Autodesk Inventor part; units mm, degrees
(part 2 of 2)
extrude "Extrusion65" cut sketch "Sketch70" against normal blind 1.5 contours L6 L7 L8 L0 | L4 L17 L14 L15
sketch "Sketch71" plane through (0, 1.5, 0) normal (0, 1, 0) x (1, 0, 0)
  line L0 (6.4642, -4.9) -> (13.4642, -4.9) projected
  line L1 (-3.6078, -4.9) -> (3.3922, -4.9) projected
  line L2 (-3.6078, -3.9) -> (3.3922, -3.9)
  line L3 (6.4642, -3.9) -> (13.4642, -3.9)
  line L4 (-3.4042, -4.9) -> (3.3922, -4.9)
  line L5 (13.4642, -4.9) -> (6.4642, -4.9)
  line L6 (6.4642, -4.9) -> (6.4642, -3.9)
  line L7 (13.4642, -4.9) -> (13.4642, -3.9)
  line L8 (6.4642, -4.9) -> (6.4642, -3.9)
  line L9 (13.4642, -4.9) -> (6.4642, -4.9)
  line L10 (3.3922, -3.9) -> (3.3922, -4.9)
  line L11 (3.3922, -4.9) -> (-3.6078, -4.9)
  line L12 (-3.6078, -4.9) -> (-3.6078, -3.9)
  point P0 (3.3922, -22.9)
  point P1 (0, 0)
  dimension "d349" = 7
  dimension "d351" = 7
  constraints: 22 end point, 4 collinear, 1 point on line
  measures "d349" distance of L2.start L2.end
  measures "d351" distance of L3.start L3.end
extrude "Extrusion66" cut sketch "Sketch71" against normal blind 1.5
sketch "Sketch75" plane through (0, 1.5, 0) normal (0, 1, 0) x (1, 0, 0)
  line L0 (-14, 20) -> (14, 20) projected
  line L1 (-14, 20) -> (0, 20)
  line L2 (0, 20) -> (0, 11.7)
  line L3 (0, 11.7) -> (-11.6, 11.7)
  line L4 (-11.6, 11.7) -> (12, 11.7)
  line L5 (12, 11.7) -> (12, -0.7)
  line L6 (12, -0.7) -> (-11.6, -0.7)
  line L7 (-11.6, -0.7) -> (-11.6, 11.7)
  point P0 (0, 0)
  dimension "d359" = 8.3
  dimension "d360" = 11.6
  dimension "d361" = 23.6
  dimension "d362" = 12.4
  constraints: 14 end point, 3 perpendicular, 2 parallel, 1 horizontal, 1 midpoint
  measures "d359" distance of L1.end L2.end
  measures "d360" distance of L2.end L3.end
  measures "d361" distance of L5.end L6.end
  measures "d362" distance of L4.end L5.end
extrude "Extrusion67" cut sketch "Sketch75" against normal blind 1.5
sketch "Sketch76" plane through (0, 1.5, 0) normal (0, 1, 0) x (1, 0, 0)
  line L0 (-11.6, -0.7) -> (-11.6, 11.7) projected
  circle A0 centre (13.95, 5.5) radius 1.5 projected
  circle A1 centre (-13.95, 5.5) radius 1.5 projected
  line L1 (6.4642, -3.9) -> (13.4642, -3.9) projected
  line L2 (-13.95, 5.5) -> (13.95, 5.5)
  line L3 (-11.6, 11.7) -> (-12, 11.7)
  line L4 (-12, 11.7) -> (-12, -0.7)
  line L5 (-12, -0.7) -> (-11.6, -0.7)
  line L6 (-11.6, 11.7) -> (-11.6, -0.7)
  point P0 (0, 0)
  dimension "d365" = 27.9
  dimension "d366" = 0.4
  constraints: 10 end point, 3 parallel, 2 perpendicular
  measures "d365" distance of L2.start L2.end
  measures "d366" distance of L0.end L3.end
extrude "Extrusion68" cut sketch "Sketch76" against normal blind 1.5 contours L5 L4 L2 L0 | L2 L4 L3 L0
sketch "Sketch77" plane through (0, 1.5, 0) normal (0, 1, 0) x (1, 0, 0)
  line L0 (-12, 11.7) -> (12, 11.7) projected
  line L1 (12, -0.7) -> (-12, -0.7) projected
  line L2 (-12, -0.7) -> (-12, 11.7) projected
  line L3 (-12, 11.7) -> (-12, -0.7)
  line L4 (-12, -0.7) -> (-11.7, -0.7)
  line L5 (-11.7, -0.7) -> (-11.7, 11.7)
  line L6 (-12, 11.7) -> (-11.7, 11.7)
  line L7 (12, 11.7) -> (12, -0.7)
  line L8 (12, -0.7) -> (11.7, -0.7)
  line L9 (11.7, -0.7) -> (11.7, 11.7)
  line L10 (11.7, 11.7) -> (12, 11.7)
  point P0 (0, 0)
  dimension "d370" = 0.3
  dimension "d371" = 0.3
  constraints: 16 end point, 5 perpendicular, 4 point on line, 1 collinear
  measures "d370" distance of L1.end L4.end
  measures "d371" distance of L1.start L8.end
extrude "Extrusion69" add sketch "Sketch77" against normal blind 1.5 contours L0 L5 L1 L2 | L0 L7 L1 L9
sketch "Sketch78" plane through (-17.5932, 0, 25.4) normal (0, 0, 1) x (1, 0, 0)
  line L0 (0, 11.5) -> (35.1864, 11.5) projected
  line L1 (17.5932, 11.5) -> (17.5932, 6.5)
  circle A0 centre (17.5932, 6.5) radius 2.5
  point P0 (17.5932, 0)
  dimension "d374" = 5
  dimension "d375" = 5
  constraints: 2 end point, 1 centre point, 1 coincident, 1 midpoint, 1 perpendicular
  measures "d374" distance of L1.start L1.end
  measures "d375" diameter of A0
extrude "Extrusion70" cut sketch "Sketch78" against normal blind 1.5
sketch "Sketch79" plane through (-17.5932, 0, 25.4) normal (0, 0, 1) x (1, 0, 0)
  circle A0 centre (17.5932, 6.5) radius 2.5 projected
  line L0 (0, 11.5) -> (35.1864, 11.5) projected
  line L1 (17.5932, 6.5) -> (11.2932, 6.5)
  line L2 (11.2932, 6.5) -> (23.8932, 6.5)
  circle A1 centre (11.2932, 6.5) radius 1.5
  circle A2 centre (23.8932, 6.5) radius 1.5
  point P0 (17.5932, 0)
  dimension "d378" = 6.3
  dimension "d379" = 12.6
  dimension "d380" = 3
  dimension "d381" = 3
  constraints: 4 end point, 2 centre point, 2 coincident, 1 collinear, 1 parallel
  measures "d378" distance of L1.start L1.end
  measures "d379" distance of L1.end L2.end
  measures "d380" diameter of A1
  measures "d381" diameter of A2
extrude "Extrusion71" cut sketch "Sketch79" against normal blind 1.5 contours A1 | A2
sketch "Sketch80" plane through (0, 0, 0) normal (0, -1, 0) x (1, 0, 0)
  line L0 (-3.6078, 3.9) -> (-3.6078, 22.9) projected
  line L1 (-3.6078, 22.9) -> (3.3922, 22.9) projected
  line L2 (3.3922, 22.9) -> (3.3922, 3.9) projected
  line L3 (3.3922, 3.9) -> (-3.6078, 3.9) projected
  line L4 (13.4642, 22.9) -> (13.4642, 3.9) projected
  line L5 (13.4642, 3.9) -> (6.4642, 3.9) projected
  line L6 (6.4642, 3.9) -> (6.4642, 22.9) projected
  line L7 (6.4642, 22.9) -> (13.4642, 22.9) projected
  point P0 (0, 0)
extrude "Extrusion72" add sketch "Sketch80" against normal blind 2
sketch "Sketch81" plane through (0, 1.5, 0) normal (0, 1, 0) x (1, 0, 0)
  line L0 (-11.7, 11.7) -> (11.7, 11.7) projected
  line L1 (11.7, 11.7) -> (11.7, -0.7) projected
  line L2 (11.7, -0.7) -> (-11.7, -0.7) projected
  line L3 (-11.7, -0.7) -> (-11.7, 11.7) projected
  line L4 (-3.6078, -22.9) -> (-3.6078, -3.9) projected
  line L5 (-3.6078, -3.9) -> (3.3922, -3.9) projected
  line L6 (3.3922, -3.9) -> (3.3922, -22.9) projected
  line L7 (3.3922, -22.9) -> (-3.6078, -22.9) projected
  circle A0 centre (-12.72, 16.04) radius 1.5 projected
  circle A1 centre (-21.72, 4.04) radius 1.5 projected
  circle A2 centre (21.72, 4.04) radius 1.5 projected
  circle A3 centre (12.72, 16.04) radius 1.5 projected
  circle A4 centre (13.95, 5.5) radius 1.5 projected
  circle A5 centre (-13.95, 5.5) radius 1.5 projected
  line L8 (-17.5932, -23.9) -> (17.5932, -23.9) projected
  line L9 (17.5932, -23.9) -> (17.5932, -11.7729) projected
  arc A6 (26, 4) -> (17.5932, -11.7729) centre (36.5932, -11.7729) ccw projected
  line L10 (14, 20) -> (26, 4) projected
  line L11 (-14, 20) -> (14, 20) projected
  line L12 (-26, 4) -> (-14, 20) projected
  arc A7 (-17.5932, -11.7729) -> (-26, 4) centre (-36.5932, -11.7729) ccw projected
  line L13 (-17.5932, -23.9) -> (-17.5932, -11.7729) projected
  line L14 (13.4642, -3.9) -> (13.4642, -22.9) projected
  line L15 (13.4642, -22.9) -> (6.4642, -22.9) projected
  line L16 (6.4642, -22.9) -> (6.4642, -3.9) projected
  line L17 (6.4642, -3.9) -> (13.4642, -3.9) projected
  point P0 (0, 0)
extrude "Extrusion73" add sketch "Sketch81" along normal blind 0.5
sketch "Sketch82" plane through (0, 11.5, 0) normal (0, 1, 0) x (1, 0, 0)
  point P0 (0, 0)
sketch "Sketch83" plane through (-17.5932, 0, 25.4) normal (0, 0, 1) x (1, 0, 0)
  circle A0 centre (11.2932, 6.5) radius 1.5 projected
  circle A1 centre (23.8932, 6.5) radius 1.5 projected
  circle A2 centre (17.5932, 6.5) radius 2.5 projected
  line L0 (0, 0) -> (0, 11.5) projected
  line L1 (35.1864, 0) -> (0, 0) projected
  line L2 (35.1864, 0) -> (35.1864, 11.5) projected
  line L3 (0, 11.5) -> (35.1864, 11.5) projected
  point P0 (17.5932, 0)
extrude "Extrusion74" add sketch "Sketch83" along normal blind 0.5
sketch "Sketch84" plane through (0, 2, 0) normal (0, 1, 0) x (1, 0, 0)
  line L0 (17.5932, -23.9) -> (-17.5932, -23.9) projected
  line L1 (-17.5932, -11.7729) -> (-17.5932, -23.9) projected
  line L2 (0, -23.9) -> (0, -20.9)
  line L3 (17.5932, -23.9) -> (13.0932, -23.9)
  line L4 (13.0932, -23.9) -> (13.0932, -20.9)
  line L5 (-17.5932, -23.9) -> (-13.0932, -23.9)
  line L6 (-13.0932, -23.9) -> (-13.0932, -20.9)
  circle A0 centre (13.0932, -20.9) radius 1.5
  circle A1 centre (0, -20.9) radius 2
  circle A2 centre (-13.0932, -20.9) radius 1.5
  line L7 (13.0932, -20.9) -> (13.0932, -5.9)
  line L8 (0, -20.9) -> (0, -5.9)
  line L9 (-13.0932, -20.9) -> (-13.0932, -5.9)
  circle A3 centre (0, -5.9) radius 2
  circle A4 centre (13.0932, -5.9) radius 1.5
  circle A5 centre (-13.0932, -5.9) radius 1.5
  line L10 (14.5932, -20.9) -> (14.5932, -5.9)
  line L11 (11.5932, -20.9) -> (11.5932, -5.9)
  line L12 (2, -20.9) -> (2, -5.9)
  line L13 (-2, -20.9) -> (-2, -5.9)
  line L14 (-11.5932, -20.9) -> (-11.5932, -5.9)
  line L15 (-14.5932, -20.9) -> (-14.5932, -5.9)
  point P0 (0, 0)
  dimension "d390" = 3
  dimension "d391" = 4.5
  dimension "d392" = 3
  dimension "d393" = 4.5
  dimension "d394" = 3
  dimension "d395" = 3
  dimension "d396" = 4
  dimension "d397" = 3
  dimension "d398" = 15
  dimension "d399" = 15
  dimension "d400" = 15
  dimension "d401" = 4
  dimension "d402" = 3
  dimension "d403" = 3
  constraints: 28 end point, 12 point on circle, 6 centre point, 6 coincident, 6 parallel, 6 tangent, 2 perpendicular, 2 point on line, 1 midpoint
  measures "d390" distance of L2.start L2.end
  measures "d391" distance of L0.start L3.end
  measures "d392" distance of L3.end L4.end
  measures "d393" distance of L0.end L5.end
  measures "d394" distance of L5.end L6.end
  measures "d395" diameter of A0
  measures "d396" diameter of A1
  measures "d397" diameter of A2
  measures "d398" distance of L7.start L7.end
  measures "d399" distance of L8.start L8.end
  measures "d400" distance of L9.start L9.end
  measures "d401" diameter of A3
  measures "d402" diameter of A4
  measures "d403" diameter of A5
extrude "Extrusion75" cut sketch "Sketch84" against normal blind 2
body "Solid1"
